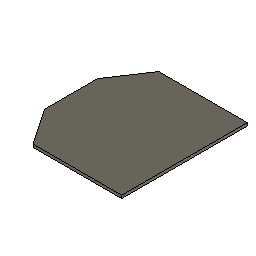
blank (Autodesk Fusion 360 design; units mm, degrees)
Autodesk Fusion 360 part; units mm, degrees
sketch "Sketch1" plane through (0, 0, 0) normal (0, 0, 1) x (1, 0, 0)
  line L0 (6.47, -5.82) -> (-6.47, -5.82)
  line L1 (-6.47, -5.82) -> (-6.47, 5.82)
  line L2 (-6.47, 5.82) -> (6.47, 5.82)
  line L3 (6.47, 5.82) -> (6.47, -5.82)
  line L4 (6.47, -5.82) -> (-6.47, 5.82) construction
  line L5 (-6.47, -5.82) -> (6.47, 5.82) construction
  line L6 (6.47, -5.82) -> (-6.47, -5.82)
  line L7 (-6.47, -5.82) -> (-6.47, 3.338)
  line L8 (-6.47, 3.338) -> (6.47, 3.338)
  line L9 (6.47, 3.338) -> (6.47, -5.82)
  line L10 (6.47, 3.338) -> (-6.47, 3.338)
  line L11 (-6.47, 3.338) -> (-6.47, -2.13)
  line L12 (-6.47, -2.13) -> (6.47, -2.13)
  line L13 (6.47, -2.13) -> (6.47, 3.338)
  line L14 (6.47, -5.82) -> (-2.649, -5.82)
  line L15 (-2.649, -5.82) -> (-2.649, 5.82)
  line L16 (-2.649, 5.82) -> (6.47, 5.82)
  line L17 (6.47, 5.82) -> (6.47, -5.82)
  line L18 (-2.649, -5.82) -> (-5.17, -5.82)
  line L19 (-5.17, -5.82) -> (-5.17, -2.13)
  line L20 (-5.17, -2.13) -> (-2.649, -2.13)
  line L21 (-2.649, -2.13) -> (-2.649, -5.82)
  line L22 (-2.649, 3.338) -> (-5.17, 3.338)
  line L23 (-5.17, 3.338) -> (-5.17, 5.82)
  line L24 (-5.17, 5.82) -> (-2.649, 5.82)
  line L25 (-2.649, 5.82) -> (-2.649, 3.338)
  line L26 (6.47, -5.82) -> (-5.17, -5.82)
  line L27 (-5.17, -5.82) -> (-5.17, 7.12)
  line L28 (-5.17, 7.12) -> (6.47, 7.12)
  line L29 (6.47, 7.12) -> (6.47, -5.82)
  line L30 (-2.649, 5.82) -> (-2.649, 7.12)
  line L31 (-2.649, 7.12) -> (-5.17, 3.338)
  line L32 (-5.17, -2.13) -> (-2.649, -5.82)
  dimension "d1" = 12.94
  dimension "d2" = 11.64
  dimension "d3" = 9.158
  dimension "d4" = 5.468
  dimension "d5" = 9.119
  dimension "d6" = 2.521
  dimension "d7" = 2.521
  dimension "d8" = 12.94
  constraint horizontal L0
  constraint perpendicular L0 L1
  constraint parallel L0 L2
  constraint parallel L1 L3
  constraint coincident L4 origin
  constraint coincident L5 origin
  constraint horizontal L6
  constraint vertical L7
  constraint horizontal L8
  constraint vertical L9
  constraint coincident L1 L7.end
  constraint horizontal L10
  constraint vertical L11
  constraint horizontal L12
  constraint vertical L13
  constraint coincident L7 L11.end
  constraint horizontal L14
  constraint vertical L15
  constraint horizontal L16
  constraint vertical L17
  constraint coincident L2 L15.end
  constraint horizontal L18
  constraint vertical L19
  constraint horizontal L20
  constraint vertical L21
  constraint coincident L12 L19.end
  constraint horizontal L22
  constraint vertical L23
  constraint horizontal L24
  constraint vertical L25
  constraint coincident L2 L23.end
  constraint coincident L15 L22.start
  constraint coincident L10 L22.start
  constraint horizontal L26
  constraint vertical L27
  constraint horizontal L28
  constraint vertical L29
  constraint coincident L28 L30.end
  constraint perpendicular L28 L30
  measures "d1" distance of L1.end L2.end
  measures "d2" distance of L0.end L1.end
  measures "d3" distance of L0.start L8.end
  measures "d4" distance of L8.end L12.end
  measures "d5" distance of L0.start L14.end
  measures "d6" distance of L14.end L18.end
  measures "d7" distance of L22.start L22.end
  measures "d8" distance of L0.start L28.end
extrude "Extrude1" add sketch "Sketch1" along normal blind 0.1 contours L0 L3 L6 L9 L12 L14 L15 L17 L21 L26 L29 | L12 L15 L20 L21 L32 | L3 L8 L9 L10 L12 L13 L15 L17 L29 | L8 L10 L12 L15 L20 L22 L27 | L2 L3 L8 L10 L15 L16 L17 L25 L29 | L2 L8 L10 L15 L22 L24 L25 L31 | L2 L16 L28 L29 L30 | L2 L24 L30 L31
extrude "Extrude2" add 1 faces at (-1.29, 1.5153, 0.1) along direction (0, 0, 1) blind 0.2
